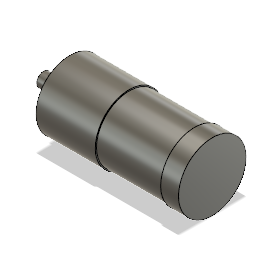
Motor (Autodesk Fusion 360 design; units mm, degrees)
Autodesk Fusion 360 part; units mm, degrees
sketch "Sketch1" plane through (0, 0, 0) normal (1, 0, 0) x (0, 0, -1)
  circle A0 centre (0, 0) radius 28.5
  dimension "d1" = 57
  measures "d1" diameter of A0
extrude "Extrude1" add sketch "Sketch1" along normal blind 15
sketch "Sketch2" plane through (0, 0, 0) normal (1, 0, 0) x (0, 0, -1)
  circle A0 centre (0, 0) radius 27.5
  dimension "d4" = 55
  measures "d4" diameter of A0
extrude "Extrude2" add sketch "Sketch2" against normal blind 55
sketch "Sketch3" plane through (-55, 0, 0) normal (-1, 0, 0) x (0, 0, 1)
  circle A0 centre (0, 0) radius 27.5
  circle A1 centre (0, 0) radius 28.5
extrude "Extrude3" add sketch "Sketch3" along normal blind 5 contours A0 | A1
sketch "Sketch4" plane through (-60, 0, 0) normal (-1, 0, 0) x (0, 0, 1)
  circle A0 centre (0, 0) radius 28.5
  circle A1 centre (0, 0) radius 28.5
extrude "Extrude4" add sketch "Sketch4" along normal blind 45
sketch "Sketch5" plane through (-105, 0, 0) normal (-1, 0, 0) x (0, 0, 1)
  circle A0 centre (0, 0) radius 28.5
  circle A1 centre (0, 0) radius 15.9875
  dimension "d11" = 31.975
  measures "d11" diameter of A1
extrude "Extrude5" add sketch "Sketch5" along normal blind 2 contours A1
sketch "Sketch6" plane through (-107, 0, 0) normal (-1, 0, 0) x (0, 0, 1)
  circle A0 centre (0, 0) radius 15.9875
  circle A1 centre (0, 0) radius 5.9925
  dimension "d14" = 11.985
  measures "d14" diameter of A1
extrude "Extrude6" add sketch "Sketch6" along normal blind 20 contours A1
sketch "Sketch7" plane through (-127, 0, 0) normal (-1, 0, 0) x (0, 0, 1)
  circle A0 centre (0, 0) radius 5.9925
  circle A1 centre (0, 0) radius 2
  dimension "d17" = 4
  measures "d17" diameter of A1
extrude "Extrude7" cut sketch "Sketch7" against normal blind 15 contours A1
equation "d11 = 32 mm - 0.025 mm"
equation "d14 = 12 mm - 0.015 mm"
